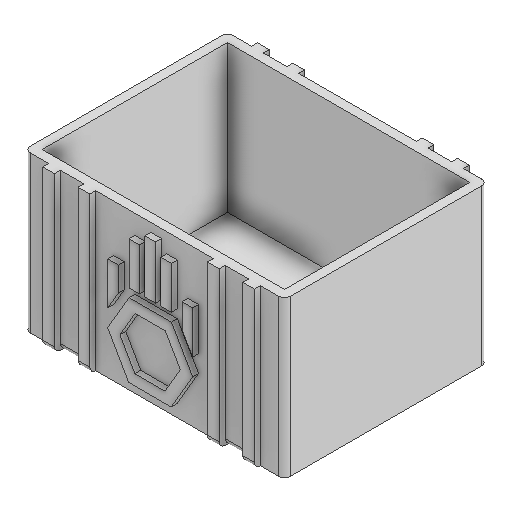
# Autodesk Inventor part: Janus wire holder
Saved by Autodesk Inventor 2025.1 (Build 291241020, 241B)
## iProperties
Created: 2025-03-14
Part Number: Janus wire holder
Material: Generic
Document SubType Name: Modeling
Designer: alexa
Density: 1 g/cm^3
Appearance: Default
Author: alexa
Autodesk Inventor part; units mm, degrees
ref_plane "YZ Plane" through (0, 0, 0) normal (1, 0, 0) x (0, 1, 0)
ref_plane "XZ Plane" through (0, 0, 0) normal (0, 1, 0) x (-1, 0, 0)
sketch "Sketch1" plane through (0, 0, 0) normal (0, 0, 1) x (1, 0, 0)
  line L0 (0, 0) -> (112.268, 0)
  line L1 (112.268, 0) -> (112.268, 67.31)
  line L2 (112.268, 67.31) -> (0, 67.31)
  line L3 (0, 67.31) -> (0, 0)
  dimension "d0" = 112.268
  dimension "d1" = 67.31
  constraints: 8 end point, 2 parallel, 1 horizontal, 1 perpendicular
  measures "d0" distance of L1.end L2.end
  measures "d1" distance of L0.end L1.end
extrude "Extrusion1" add sketch "Sketch1" along normal blind 87.63
shell "Shell1" thickness 3.81 removed faces 1 at (74.8453, 67.31, 29.21)
sketch "Sketch2" plane through (0, 0, 87.63) normal (0, 0, 1) x (1, 0, 0)
  line L0 (112.268, 67.31) -> (0, 67.31) projected
  line L1 (0, 0) -> (112.268, 0) projected
  line L2 (10.414, 67.31) -> (15.494, 67.31)
  line L3 (15.494, 67.31) -> (15.494, 0)
  line L4 (15.494, 0) -> (10.414, 0)
  line L5 (10.414, 0) -> (10.414, 67.31)
  line L6 (25.654, 0) -> (30.734, 0)
  line L7 (30.734, 0) -> (30.734, 67.31)
  line L8 (30.734, 67.31) -> (25.654, 67.31)
  line L9 (25.654, 67.31) -> (25.654, 0)
  line L10 (86.614, 67.31) -> (81.534, 67.31)
  line L11 (81.534, 67.31) -> (81.534, 0)
  line L12 (81.534, 0) -> (86.614, 0)
  line L13 (86.614, 0) -> (86.614, 67.31)
  line L14 (96.774, 0) -> (101.854, 0)
  line L15 (101.854, 0) -> (101.854, 67.31)
  line L16 (101.854, 67.31) -> (96.774, 67.31)
  line L17 (96.774, 67.31) -> (96.774, 0)
  point P0 (56.134, 0)
  dimension "d5" = 5.08
  dimension "d6" = 5.08
  dimension "d7" = 5.08
  dimension "d8" = 5.08
  dimension "d9" = 10.16
  dimension "d10" = 10.16
  dimension "d11" = 50.8
  dimension "d12" = 25.4
  constraints: 32 end point, 8 parallel, 8 point on line, 4 horizontal, 4 perpendicular, 1 midpoint
  measures "d5" distance between parallel lines of L13 L11
  measures "d6" distance between parallel lines of L15 L17
  measures "d7" distance between parallel lines of L7 L9
  measures "d8" distance between parallel lines of L3 L5
  measures "d9" distance between parallel lines of L9 L3
  measures "d10" distance between parallel lines of L17 L13
  measures "d11" distance between parallel lines of L11 L7
  measures "d12" distance from line of point (56.134, 0) L7
extrude "Extrusion2" add sketch "Sketch2" along normal blind 2.54 contours L15 L1 L17 L0 | L13 L1 L11 L0 | L7 L1 L9 L0 | L3 L1 L5 L0
ref_plane "Work Plane1" through (0, 0, 43.815) normal (0, 0, 1) x (1, 0, 0)
mirror "Mirror1" about plane through (0, 0, 43.815) normal (0, 0, 1) of "Extrusion2"
fillet "Fillet1" radius 2.54 12 edges at (12.954, 0, 90.17) (28.194, 0, 90.17) (20.574, 0, 87.63) (84.074, 0, 90.17) (91.694, 0, 87.63) (99.314, 0, 90.17) (12.954, 0, -2.54) (20.574, 0, 0) (28.194, 0, -2.54) (91.694, 0, 0) (99.314, 0, -2.54) (84.074, 0, -2.54)
sketch "Sketch3" plane through (0, 0, 87.63) normal (0, 0, 1) x (1, 0, 0)
  line L0 (65.8267, 5.2092) -> (47.5136, 5.3082)
  line L1 (47.5136, 5.3082) -> (38.4421, 21.2186)
  line L2 (38.4421, 21.2186) -> (47.6874, 37.0338)
  line L3 (47.6874, 37.0338) -> (65.9845, 37.0338)
  line L4 (65.9845, 37.0338) -> (75.1503, 21.1582)
  line L5 (75.1503, 21.1582) -> (65.8267, 5.2092)
  line L6 (50.3144, 32.4551) -> (43.729, 21.19)
  line L7 (43.729, 21.19) -> (50.1818, 9.8726)
  line L8 (50.1818, 9.8726) -> (63.208, 9.8021)
  line L9 (63.208, 9.8021) -> (69.855, 21.1725)
  line L10 (69.855, 21.1725) -> (63.341, 32.4551)
  line L11 (63.341, 32.4551) -> (50.3144, 32.4551)
  line L12 (38.5123, 28.5967) -> (38.5123, 46.9115)
  line L13 (38.5123, 46.9115) -> (43.091, 46.9115)
  line L14 (43.091, 46.9115) -> (43.091, 36.4292)
  line L15 (43.091, 36.4292) -> (38.5123, 28.5967)
  line L16 (47.6697, 59.0116) -> (52.2484, 59.0116)
  line L17 (52.2484, 59.0116) -> (52.2484, 40.6967)
  line L18 (65.9845, 40.6967) -> (65.9845, 59.0116)
  line L19 (65.9845, 59.0116) -> (61.4058, 59.0116)
  line L20 (61.4058, 59.0116) -> (61.4058, 40.6967)
  line L21 (75.1419, 28.4986) -> (75.1419, 46.9115)
  line L22 (75.1419, 46.9115) -> (70.5632, 46.9115)
  line L23 (70.5632, 46.9115) -> (70.5632, 36.4292)
  line L24 (70.5632, 36.4292) -> (75.1419, 28.4986)
  line L25 (54.5377, 63.5903) -> (54.5377, 40.6967)
  line L26 (54.5377, 40.6967) -> (59.1164, 40.6967)
  line L27 (59.1164, 40.6967) -> (59.1164, 63.5903)
  line L28 (59.1164, 63.5903) -> (54.5377, 63.5903)
  line L29 (61.4058, 40.6967) -> (65.9845, 40.6967)
  line L30 (52.2484, 59.0116) -> (54.5377, 59.0116) construction
  line L31 (61.4058, 59.0116) -> (59.1164, 59.0116) construction
  line L32 (47.6697, 59.0116) -> (47.6697, 40.6967)
  line L33 (47.6697, 40.6967) -> (52.2484, 40.6967)
  line L34 (81.534, 67.31) -> (81.534, 2.54) projected
  point P0 (0, 0)
  point P1 (56.3847, 20.5734)
  point P2 (56.6949, 9.8373)
  dimension "d16" = 18.3134
  dimension "d17" = 4.5787
  dimension "d18" = 3.663
  dimension "d19" = 3.663
  dimension "d20" = 4.5787
  dimension "d21" = 4.5787
  dimension "d22" = 4.5787
  dimension "d23" = 4.5787
  dimension "d24" = 3.663
  dimension "d25" = 18.3148
  dimension "d26" = 18.3148
  dimension "d27" = 22.8935
  dimension "d28" = 4.5787
  dimension "d29" = 4.5787
  dimension "d30" = 4.5787
  dimension "d31" = 2.2894
  dimension "d32" = -4.5964
  dimension "d33" = 24.8391
  constraints: 68 end point, 8 perpendicular, 7 point on line, 5 parallel, 3 collinear, 1 midpoint, 6 other
  measures "d16" distance of L0.start L0.end
  measures "d17" distance between parallel lines of L2 L6
  measures "d18" distance between parallel lines of L15 L2
  measures "d19" distance between parallel lines of L24 L4
  measures "d20" distance between parallel lines of L14 L12
  measures "d21" distance between parallel lines of L21 L23
  measures "d22" distance between parallel lines of L18 L20
  measures "d23" distance between parallel lines of L25 L27
  measures "d24" distance between parallel lines of L33 L3
  measures "d25" distance between parallel lines of L16 L33
  measures "d26" distance from line of L13 L15.end
  measures "d27" distance between parallel lines of L28 L26
  measures "d28" distance between parallel lines of L32 L17
  measures "d29" distance between parallel lines of L32 L14
  measures "d30" distance between parallel lines of L23 L18
  measures "d31" distance between parallel lines of L27 L20
  measures "d32" horizontal distance of L2.end L15.start
  measures "d33" distance from line of L34 point (56.695, 9.837)
extrude "Extrusion3" add sketch "Sketch3" along normal blind 2.54
fillet "Fillet2" radius 2.54 4 edges at (0, 33.655, 87.63) (112.268, 33.655, 87.63) (112.268, 33.655, 0) (0, 33.655, 0)
equation "\"d5\" = d6"
equation "\"d7\" = d6"
equation "\"d8\" = d7"
equation "\"d10\" = d9"
body "Solid1"
